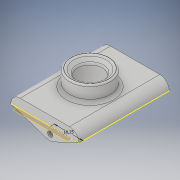
# Autodesk Inventor part: support
Saved by Autodesk Inventor 2019 (Build 230136000, 136)
## iProperties
Created: 2021-11-08
Part Number: support
Material: Genérico
Document SubType Name: Modeling
Designer: Juan M. Casillas
Density: 1 g/cm^3
Appearance: Valor por defecto
Author: Juan M. Casillas
Autodesk Inventor part; units mm, degrees
ref_plane "YZ Plane" through (0, 0, 0) normal (1, 0, 0) x (0, 1, 0)
ref_plane "XZ Plane" through (0, 0, 0) normal (0, 1, 0) x (-1, 0, 0)
ref_plane "XY Plane" through (0, 0, 0) normal (0, 0, 1) x (1, 0, 0)
sketch "Sketch1" plane through (0, 0, 0) normal (0, 1, 0) x (-1, 0, 0)
  line L0 (21.75, 28.875) -> (-21.75, 28.875)
  line L1 (-21.75, 28.875) -> (-21.75, -28.875)
  line L2 (-21.75, -28.875) -> (21.75, -28.875)
  line L3 (21.75, -28.875) -> (21.75, 28.875)
  line L4 (21.75, 28.875) -> (-21.75, -28.875) construction
  line L5 (-21.75, 28.875) -> (21.75, -28.875) construction
  point P0 (0, 0)
  dimension "d0" = 43.5
  dimension "d1" = 57.75
  constraints: 12 end point, 2 midpoint, 2 parallel, 1 horizontal, 1 perpendicular
  measures "d0" distance of L2.end L1.end
  measures "d1" distance of L1.end L0.end
extrude "Extrusion1" add sketch "Sketch1" along normal blind 6
fillet "Fillet1" radius 6 1 edges at (21.75, 6, 0)
fillet "Fillet2" radius 6 1 edges at (-21.75, 6, 0)
sketch "Sketch2" plane through (0, 0, 0) normal (0, -1, 0) x (1, 0, 0)
  line L0 (-21.75, 28.875) -> (21.75, 28.875) projected
  line L1 (-21.75, -28.875) -> (-21.75, 28.875) projected
  line L2 (21.75, -28.875) -> (-21.75, -28.875) projected
  line L3 (21.75, 28.875) -> (21.75, -28.875) projected
  line L4 (21.75, 28.875) -> (21.75, -28.875) construction
  line L5 (21.75, 28.875) -> (3.5, 28.875) construction
  line L6 (-21.75, 28.875) -> (21.75, 28.875) construction
  point P0 (0, 0)
  dimension "d6" = 18.25
  constraints: 2 end point, 1 point on line
  measures "d6" distance of L0.end L5.end
extrude "Extrusion2" add sketch "Sketch2" along normal blind 8.5
sketch "Sketch3" plane through (-15.75, 6, 28.875) normal (0, 0, 1) x (1, 0, 0)
  arc A0 (0, 0) -> (-6, -6) centre (0, -6) ccw construction
  line L0 (-6, -6) -> (-6, -14.5) construction
  line L1 (37.5, -14.5) -> (-6, -14.5) construction
  line L2 (37.5, -6) -> (37.5, -14.5) construction
  arc A1 (37.5, -6) -> (31.5, 0) centre (31.5, -6) ccw construction
  line L3 (0, 0) -> (31.5, 0) construction
  line L4 (19.1951, -6) -> (19.1951, -10.25) construction
  point P0 (15.75, -6)
  dimension "d9" = 4.25
  constraints: 2 end point, 1 coincident, 1 vertical
  measures "d9" distance of L4.start L4.end
hole "Hole1" at (3.4451, -4.25, 28.875) direction (0, 0, -1) diameter 3.3 end through all
sketch "Sketch4" plane through (-15.75, 6, 28.875) normal (0, 0, 1) x (1, 0, 0)
  circle A0 centre (19.1951, -10.25) radius 1.65 construction
  line L0 (19.1951, -10.25) -> (19.1951, -14.5) construction
  line L1 (-6, -14.5) -> (37.5, -14.5) construction
  line L2 (37.5, -6) -> (37.5, -14.5) projected
  line L3 (19.1951, -14.5) -> (37.5, -6)
  line L4 (-6, -6) -> (-6, -14.5) projected
  line L5 (19.1951, -14.5) -> (-6, -6)
  line L6 (-6, -6) -> (-6, -14.5)
  line L7 (19.1951, -14.5) -> (37.5, -14.5)
  line L8 (37.5, -14.5) -> (37.5, -6)
  line L9 (19.1951, -14.5) -> (-6, -14.5)
  point P0 (15.75, -6)
  constraints: 14 end point, 4 collinear, 1 point on line, 1 vertical
extrude "Extrusion3" cut sketch "Sketch4" against normal through all
fillet "Fillet3" radius 6 1 edges at (3.4451, -8.5, 0)
ref_plane "Work Plane1" through (0, 0, 0) normal (0, 1, 0) x (1, 0, 0)
sketch "Sketch5" plane through (0, 0, 0) normal (0, 1, 0) x (1, 0, 0)
  line L0 (21.75, -28.875) -> (21.75, 28.875) projected
  line L1 (-21.75, 28.875) -> (-21.75, -28.875) projected
  line L2 (21.75, -23.875) -> (-21.75, -23.875)
  line L3 (-21.75, -23.875) -> (-21.75, 23.875)
  line L4 (-21.75, 23.875) -> (21.75, 23.875)
  line L5 (21.75, 23.875) -> (21.75, -23.875)
  line L6 (21.75, -28.875) -> (15.75, -28.875) projected
  line L7 (15.75, 28.875) -> (21.75, 28.875) projected
  point P0 (0, 0)
  dimension "d21" = 5
  dimension "d22" = 5
  constraints: 8 end point, 2 parallel, 2 point on line, 1 horizontal, 1 perpendicular
  measures "d21" distance between parallel lines of L6 L2
  measures "d22" distance between parallel lines of L7 L4
extrude "Extrusion4" cut sketch "Sketch5" against normal blind 8.5
sketch "Sketch6" plane through (0, 6, 0) normal (0, 1, 0) x (1, 0, 0)
  circle A0 centre (0, 0) radius 8
  dimension "d25" = 16
  constraints: 1 centre point, 1 coincident
  measures "d25" diameter of A0
extrude "Extrusion5" cut sketch "Sketch6" against normal blind 8.5
sketch "Sketch7" plane through (0, 6, 0) normal (0, 1, 0) x (1, 0, 0)
  circle A0 centre (0, 0) radius 8 projected
  circle A1 centre (0, 0) radius 13
  dimension "d28" = 5
  constraints: 1 centre point
  measures "d28" radial gap between concentric circles of A0 A1
extrude "Extrusion6" add sketch "Sketch7" along normal blind 10
fillet "Fillet4" radius 2 1 edges at (-13, 6, 0)
chamfer "Chamfer1" distance 3 angle 45 1 edges at (-8, 16, 0)
fillet "Fillet5" radius 2 2 edges at (-11, 16, 0) (-8, 13, 0)
fillet "Fillet6" radius 1 1 edges at (-13, 16, 0)
equation "\"d22\" = d21"
body "Solid1"
